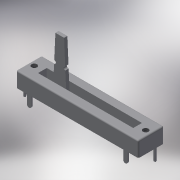
# Autodesk Inventor part: 10K Linear Pot - 737-7776
Saved by Autodesk Inventor 2017 (Build 210142000, 142)
## iProperties
Created: 2013-02-07
Part Number: 10K Linear Pot - 737-7776
Material: Generic
Document SubType Name: Modeling
Designer: chrism
Density: 1 g/cm^3
Appearance: Default
Author: chrism
Autodesk Inventor part; units mm, degrees
ref_plane "YZ Plane" through (0, 0, 0) normal (1, 0, 0) x (0, 1, 0)
ref_plane "XZ Plane" through (0, 0, 0) normal (0, 1, 0) x (-1, 0, 0)
ref_plane "XY Plane" through (0, 0, 0) normal (0, 0, 1) x (1, 0, 0)
sketch "Sketch1" plane through (0, 0, 0) normal (0, 0, 1) x (1, 0, 0)
  line L0 (-22.5, 4.7) -> (22.5, 4.7)
  line L1 (22.5, 4.7) -> (22.5, -4.7)
  line L2 (22.5, -4.7) -> (-22.5, -4.7)
  line L3 (-22.5, -4.7) -> (-22.5, 4.7)
  point P0 (0, 0)
  point P1 (-22.5, 0)
  point P2 (0, 4.7)
  dimension "d0" = 45
  dimension "d1" = 9.4
  constraints: 8 end point, 2 midpoint, 2 parallel, 1 horizontal, 1 horizontal alignment, 1 perpendicular, 1 vertical alignment
  measures "d0" distance of L0.start L0.end
  measures "d1" distance of L2.end L0.start
extrude "Extrusion1" add sketch "Sketch1" along normal blind 5.6
sketch "Sketch2" plane through (0, 0, 5.6) normal (0, 0, 1) x (1, 0, 0)
  line L0 (-22.5, 4.7) -> (22.5, 4.7) projected
  line L1 (22.5, -4.7) -> (-22.5, -4.7) projected
  line L2 (-17.5, 1.6) -> (17.5, 1.6)
  line L3 (17.5, 1.6) -> (17.5, -1.6)
  line L4 (17.5, -1.6) -> (-17.5, -1.6)
  line L5 (-17.5, -1.6) -> (-17.5, 1.6)
  point P0 (0, 0)
  dimension "d6" = 3.1
  dimension "d7" = 3.1
  dimension "d63" = 35
  dimension "d64" = 17.5
  constraints: 8 end point, 2 parallel, 1 horizontal, 1 perpendicular
  measures "d6" distance between parallel lines of L0 L2
  measures "d7" distance between parallel lines of L1 L4
  measures "d63" distance of L2.start L2.end
  measures "d64" distance from line of point (0, 0) L5
extrude "Extrusion2" cut sketch "Sketch2" against normal blind 4.3
fillet "Fillet1" radius 0.5 4 edges at (-22.5, 0, 5.6) (0, 4.7, 5.6) (22.5, 0, 5.6) (0, -4.7, 5.6)
fillet "Fillet2" radius 0.5 8 edges at (-22.3536, -4.5536, 5.4536) (-22.5, -4.7, 2.55) (-22.3536, 4.5536, 5.4536) (-22.5, 4.7, 2.55) (22.3536, 4.5536, 5.4536) (22.5, 4.7, 2.55) (22.3536, -4.5536, 5.4536) (22.5, -4.7, 2.55)
sketch "Sketch3" plane through (0, 0, 5.6) normal (0, 0, 1) x (1, 0, 0)
  circle A0 centre (-20.5, 0) radius 1
  circle A1 centre (20.5, 0) radius 1
  line L0 (-22.5, 4.2) -> (-22.5, -4.2) projected
  line L1 (22.5, -4.2) -> (22.5, 4.2) projected
  point P0 (0, 0)
  dimension "d12" = 2
  dimension "d13" = 2
  dimension "d65" = 41
  dimension "d66" = 20.5
  constraints: 2 centre point
  measures "d12" diameter of A0
  measures "d13" diameter of A1
  measures "d65" distance of A1.centre A0.centre
  measures "d66" distance of A0.centre point (0, 0)
extrude "Extrusion3" cut sketch "Sketch3" against normal blind 4
thread "Thread1" size "M2x0.4" class "6H" standard "ANSI Metric M Profile" full length
thread "Thread2" size "M2x0.4" class "6H" standard "ANSI Metric M Profile" full length
sketch "Sketch4" plane through (-22, -4.7, 0) normal (0, -1, 0) x (1, 0, 0)
  line L0 (44, 0) -> (0, 0) projected
  line L1 (40.5, 0) -> (38.9, 0)
  line L2 (38.9, 0) -> (38.9, -4)
  line L3 (38.9, -4) -> (40.5, -4)
  line L4 (40.5, -4) -> (40.5, 0)
  line L5 (3.5, 0) -> (5.1, 0)
  line L6 (5.1, 0) -> (5.1, -4)
  line L7 (5.1, -4) -> (3.5, -4)
  line L8 (3.5, -4) -> (3.5, 0)
  line L9 (44.5, 0) -> (44.5, 5.1) projected
  line L10 (-0.5, 5.1) -> (-0.5, 0) projected
  point P0 (22, 0)
  dimension "d22" = 4
  dimension "d23" = 1.6
  dimension "d24" = 4
  dimension "d25" = 4
  dimension "d26" = 1.6
  dimension "d27" = 4
  constraints: 16 end point, 4 parallel, 2 horizontal, 2 perpendicular, 2 point on line
  measures "d22" distance between parallel lines of L4 L9
  measures "d23" distance of L2.end L3.end
  measures "d24" distance of L3.end L1.start
  measures "d25" distance between parallel lines of L8 L10
  measures "d26" distance of L6.end L7.end
  measures "d27" distance of L5.end L6.end
extrude "Extrusion4" add sketch "Sketch4" against normal blind 0.5
fillet "Fillet3" radius 0.8 4 edges at (-18.5, -4.45, -4) (-16.9, -4.45, -4) (16.9, -4.45, -4) (18.5, -4.45, -4)
sketch "Sketch5" plane through (-22, 4.7, 0) normal (0, 1, 0) x (1, 0, 0)
  line L0 (0, 0) -> (44, 0) projected
  line L1 (6.1, 0) -> (4.5, 0)
  line L2 (4.5, 0) -> (4.5, 4)
  line L3 (4.5, 4) -> (6.1, 4)
  line L4 (6.1, 4) -> (6.1, 0)
  line L5 (39.5, 0) -> (37.9, 0)
  line L6 (37.9, 0) -> (37.9, 4)
  line L7 (37.9, 4) -> (39.5, 4)
  line L8 (39.5, 4) -> (39.5, 0)
  line L9 (44.5, -5.1) -> (44.5, 0) projected
  line L10 (-0.5, 0) -> (-0.5, -5.1) projected
  point P0 (22, 0)
  dimension "d31" = 1.6
  dimension "d32" = 4
  dimension "d33" = 4
  dimension "d34" = 1.6
  dimension "d35" = 5
  dimension "d36" = 5
  constraints: 16 end point, 4 parallel, 2 horizontal, 2 perpendicular, 2 point on line
  measures "d31" distance of L2.end L3.end
  measures "d32" distance of L1.end L2.end
  measures "d33" distance of L5.end L6.end
  measures "d34" distance of L6.end L7.end
  measures "d35" distance between parallel lines of L9 L8
  measures "d36" distance between parallel lines of L2 L10
extrude "Extrusion5" add sketch "Sketch5" against normal blind 0.5
fillet "Fillet4" radius 0.8 4 edges at (17.5, 4.45, -4) (15.9, 4.45, -4) (-17.5, 4.45, -4) (-15.9, 4.45, -4)
sketch "Sketch6" plane through (0, 0, 0) normal (0, 0, -1) x (-1, 0, 0)
  line L0 (-22.5, 4.2) -> (-22.5, -4.2) projected
  line L1 (22.5, -4.2) -> (22.5, 4.2) projected
  line L2 (22.5, 2.05) -> (22.1, 2.05)
  line L3 (22.1, 2.05) -> (22.1, 1.25)
  line L4 (22.1, 1.25) -> (22.5, 1.25)
  line L5 (22.5, 1.25) -> (22.5, 2.05)
  line L6 (22.5, -1.25) -> (22.1, -1.25)
  line L7 (22.1, -1.25) -> (22.1, -2.05)
  line L8 (22.1, -2.05) -> (22.5, -2.05)
  line L9 (22.5, -2.05) -> (22.5, -1.25)
  line L10 (-22.5, 2.05) -> (-22.1, 2.05)
  line L11 (-22.1, 2.05) -> (-22.1, 1.25)
  line L12 (-22.1, 1.25) -> (-22.5, 1.25)
  line L13 (-22.5, 1.25) -> (-22.5, 2.05)
  point P0 (0, 0)
  point P1 (-22.5, 1.65)
  dimension "d40" = 0.8
  dimension "d41" = 0.4
  dimension "d42" = 0.4
  dimension "d43" = 0.8
  dimension "d44" = 0.8
  dimension "d45" = 0.4
  dimension "d46" = 2.5
  dimension "d47" = 1.25
  constraints: 24 end point, 6 parallel, 3 horizontal, 3 perpendicular, 3 point on line, 1 collinear, 1 midpoint
  measures "d40" distance of L2.end L3.end
  measures "d41" distance of L2.start L2.end
  measures "d42" distance of L6.start L6.end
  measures "d43" distance of L6.end L7.end
  measures "d44" distance of L10.end L11.end
  measures "d45" distance of L10.start L10.end
  measures "d46" distance between parallel lines of L4 L6
  measures "d47" distance from line of point (0, 0) L6
extrude "Extrusion6" add sketch "Sketch6" along normal blind 4.3
fillet "Fillet5" radius 0.4 6 edges at (22.3, 2.05, -4.3) (22.3, 1.25, -4.3) (-22.3, 1.25, -4.3) (-22.3, 2.05, -4.3) (-22.3, -1.25, -4.3) (-22.3, -2.05, -4.3)
sketch "Sketch8" plane through (0, 0, 0) normal (0, 1, 0) x (-1, 0, 0)
  line L0 (-17.5, 5.6) -> (-17.5, 1.3) projected
  line L1 (17.5, 5.6) -> (17.5, 1.3) projected
  line L2 (-17.5, 5.6) -> (17.5, 5.6) projected
  line L3 (8.0304, 1.3) -> (13.0304, 1.3)
  line L4 (13.0304, 1.3) -> (12.1304, 20.6)
  line L5 (12.1304, 20.6) -> (8.9304, 20.6)
  line L6 (8.9304, 20.6) -> (8.0304, 1.3)
  line L7 (17.5, 1.3) -> (-17.5, 1.3) projected
  point P0 (0, 0)
  point P1 (10.5304, 20.6)
  point P2 (10.5304, 1.3)
  dimension "d51" = 5
  dimension "d52" = 3.2
  dimension "d53" = 15
  dimension "d62" = 35
  constraints: 8 end point, 2 midpoint, 2 parallel, 1 collinear, 1 vertical alignment
  measures "d51" distance of L3.start L3.end
  measures "d52" distance of L4.end L5.end
  measures "d53" distance between parallel lines of L2 L5
  measures "d62" distance of L1.end L0.end
extrude "Extrusion7" add sketch "Sketch8" along normal mid plane 1.2 contours L6 L5 L4 L2 | L2 L4 L3 L6
sketch "Sketch9" plane through (0, -0.6, 0) normal (0, -1, 0) x (1, 0, 0)
  line L0 (-13.0304, 1.3) -> (-12.1304, 20.6) projected
  line L1 (-8.9304, 20.6) -> (-8.0304, 1.3) projected
  line L2 (-12.1304, 20.6) -> (-8.9304, 20.6) projected
  circle A0 centre (-12.5734, 11.1) radius 0.65
  circle A1 centre (-8.4874, 11.1) radius 0.65
  point P0 (0, 0)
  dimension "d56" = 1.3
  dimension "d57" = 1.3
  dimension "d58" = 9.5
  dimension "d59" = 9.5
  constraints: 2 centre point, 2 point on line
  measures "d56" diameter of A0
  measures "d57" diameter of A1
  measures "d58" distance from line of A0.centre L2
  measures "d59" distance from line of L2 A1.centre
extrude "Extrusion8" cut sketch "Sketch9" against normal blind 1.2
equation "\"d64\" = 0.5 * d63"
equation "\"d66\" = 0.5 * d65"
equation "\"d47\" = 0.5 * d46"
equation "\"d59\" = d58"
body "Solid1"
